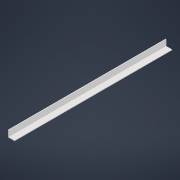
# Autodesk Inventor part: slide_panel_back_stopper
Saved by Autodesk Inventor 2021 (Build 250183000, 183)
## iProperties
Created: 2023-03-30
Part Number: slide_panel_back_stopper
Material: 一般
Document SubType Name: Modeling
Designer: casey
Density: 1 g/cm^3
Appearance: 既定
Author: casey
Autodesk Inventor part; units mm, degrees
ref_plane "YZ Plane" through (0, 0, 0) normal (1, 0, 0) x (0, 1, 0)
ref_plane "XZ Plane" through (0, 0, 0) normal (0, 1, 0) x (-1, 0, 0)
ref_plane "XY Plane" through (0, 0, 0) normal (0, 0, 1) x (1, 0, 0)
sketch "スケッチ2" plane through (0, 0, 0) normal (0, 0, 1) x (1, 0, 0)
  line L0 (0, 0) -> (15, 0)
  line L1 (15, 0) -> (15, 1)
  line L2 (15, 1) -> (0, 1)
  line L3 (0, 1) -> (0, 0)
  line L4 (0, 0) -> (1, 0)
  line L5 (1, 0) -> (1, 15)
  line L6 (1, 15) -> (0, 15)
  line L7 (0, 15) -> (0, 0)
  point P0 (1, 1)
  dimension "d0" = 15
  dimension "d1" = 1
  dimension "d2" = 1
  dimension "d3" = 15
  constraints: 16 end point, 4 parallel, 2 horizontal, 2 perpendicular
  measures "d0" distance of L2.end L1.end
  measures "d1" distance of L1.end L0.end
  measures "d2" distance of L6.end L5.end
  measures "d3" distance of L5.end L4.end
extrude "押し出し1" add sketch "スケッチ2" along normal blind 240
sketch "スケッチ3" plane through (1, 1, 0) normal (0, 1, 0) x (1, 0, 0)
  line L0 (14, 0) -> (0, 0) projected
  line L1 (0, 0) -> (0, -240) projected
  line L2 (14, 0) -> (14, -240) projected
  line L3 (14, 0) -> (14, -240) projected
  line L4 (14, -240) -> (0, -240) projected
  point P0 (-1, 0)
  point P1 (7, -233)
  point P2 (7, -120)
  point P3 (7, -7)
  point P4 (14, -120)
  dimension "d13" = 7
  dimension "d14" = 7
  dimension "d15" = 7
  dimension "d16" = 0
  dimension "d17" = 7
  dimension "d18" = 7
  constraints: 1 midpoint
  measures "d13" distance from line of L0 point (7, -7)
  measures "d14" distance from line of L1 point (7, -7)
  measures "d15" distance from line of L2 point (7, -120)
  measures "d16" vertical distance of point (7, -120) point (14, -120)
  measures "d17" distance from line of L2 point (7, -233)
  measures "d18" distance from line of L4 point (7, -233)
hole "穴1" at (8, 1, 233) at (8, 1, 120) at (8, 1, 7) direction (0, -1, 0) diameter 3.5 end through all
